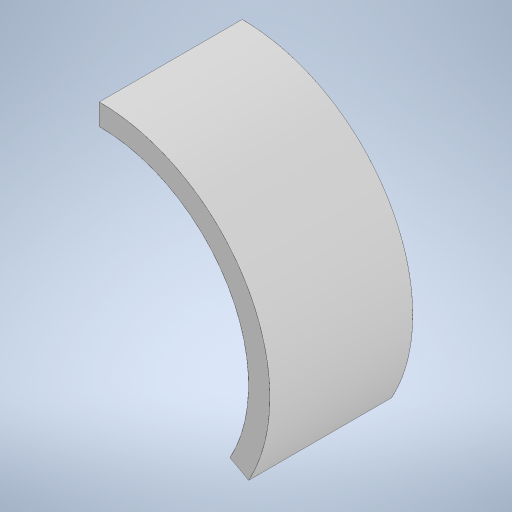
# Autodesk Inventor part: formav2
Saved by Autodesk Inventor 2024 (Build 280153000, 153)
## iProperties
Created: 2023-10-06
Part Number: formav2
Material: Ogólny
Document SubType Name: Modeling
Designer: Pawel
Density: 1 g/cm^3
Appearance: Domyślna
Author: Pawel
Autodesk Inventor part; units mm, degrees
ref_plane "YZ Plane" through (0, 0, 0) normal (1, 0, 0) x (0, 1, 0)
ref_plane "XZ Plane" through (0, 0, 0) normal (0, 1, 0) x (-1, 0, 0)
ref_plane "XY Plane" through (0, 0, 0) normal (0, 0, 1) x (1, 0, 0)
sketch "Szkic1" plane through (0, 0, 0) normal (0, 0, 1) x (1, 0, 0)
  circle A0 centre (0, 0) radius 12
  line L0 (-0.9273, 2.8531) -> (-2, 9.798)
  line L1 (0, 7) -> (0, 5.5022)
  line L2 (0.9273, 2.8531) -> (2, 9.798)
  line L3 (-1.3944, 1.0574) -> (1.3944, 1.0574)
  line L4 (-0.5425, -1.6638) -> (-1.0104, -2.8247)
  line L5 (0.5425, -1.6638) -> (1.0104, -2.8247)
  line L6 (-2.9345, -0.6234) -> (-9.4853, -3.1669)
  line L7 (-2.0072, -2.2296) -> (-7.4853, -6.631)
  line L8 (2.0072, -2.2296) -> (7.4853, -6.631)
  line L9 (2.9345, -0.6234) -> (9.4853, -3.1669)
  arc A1 (-2.0072, -2.2296) -> (-1.0104, -2.8247) centre (0, 0) ccw
  arc A2 (1.0104, -2.8247) -> (2.0072, -2.2296) centre (0, 0) ccw
  arc A3 (2.9345, -0.6234) -> (0.9273, 2.8531) centre (0, 0) ccw
  arc A4 (-0.9273, 2.8531) -> (-2.9345, -0.6234) centre (0, 0) ccw
  arc A5 (-2, 9.798) -> (-9.4853, -3.1669) centre (0, 0) ccw
  arc A6 (-7.4853, -6.631) -> (7.4853, -6.631) centre (0, 0) ccw
  arc A7 (9.4853, -3.1669) -> (2, 9.798) centre (0, 0) ccw
  arc A8 (0.5425, -1.6638) -> (1.3944, 1.0574) centre (0, 0) ccw
  arc A9 (-1.3944, 1.0574) -> (-0.5425, -1.6638) centre (0, 0) ccw
  circle A10 centre (0, 0) radius 13.5
  circle A11 centre (0, 0) radius 14.5
  line L10 (7.4853, -6.631) -> (9.4853, -3.1669)
  line L11 (11.8024, -6.5538) -> (12.6981, -7.0006)
  line L12 (11.8024, -6.5538) -> (0, 0)
  line L13 (0, 0) -> (0, 14.5)
  point P0 (-0.7322, 1.5895)
  point P1 (0.7322, 1.5895)
  point P2 (0, 13.5)
  point P3 (0, 1.0574)
  point P4 (1.5299, -0.8496)
  dimension "d2" = 360
  constraints: 28 end point, 20 point on circle, 11 centre point, 6 coincident, 2 symmetric about line, 2 vertical, 1 horizontal, 22 other
extrude "Wyciągnięcie proste2" add sketch "Szkic1" along normal blind 2 contours L2 A7 L9 A3
extrude "Wyciągnięcie proste3" add sketch "Szkic1" along normal blind 12 contours L13 A11 L11 A10 picked at (13.9327, 2.0769)
extrude "Wyciągnięcie proste4" add sketch "Szkic1" against normal blind 1 contours A0 L12 A8 L3 L13 L1 | A0 L13 A10 L12 | L13 A11 L11 A10 | L2 A7 L9 A3 picked at (12.8872, 1.0013) picked at (13.9327, 2.0769)
thicken "Pogrubienie1" operation add thickness 0.1 both sides no extend neighbours no toward (0.8451894, 0.5344669, 0) faces at (8.4519, 5.3447, 1.3333)
thicken "Pogrubienie2" operation add thickness 0.1 both sides no extend neighbours no toward (-0.3619484, -0.9321981, 0) faces at (5.1181, -1.4713, 0.6667)
thicken "Pogrubienie3" operation add thickness 0.1 both sides no extend neighbours no toward (-0.9882815, 0.1526425, 0) faces at (1.6424, 7.483, 0.6667)
sketch "Szkic2" plane through (0, 0, 0) normal (0, 0, 1) x (1, 0, 0)
  circle A0 centre (0, 0) radius 3
  constraints: 1 centre point, 1 coincident
extrude "Wyciągnięcie proste5" cut sketch "Szkic2" against normal blind 1
thicken "Pogrubienie4" operation cut thickness 1 both sides no extend neighbours no toward (0, 0, 1) faces at (7.6782, 0.304, 2)
sketch "Szkic3" plane through (0, 0, 2) normal (0, 0, 1) x (1, 0, 0)
  arc A0 (2.9345, -0.6234) -> (0.9273, 2.8531) centre (0, 0) ccw projected
  circle A1 centre (0, 0) radius 11.4018
  point P0 (0, 0)
  constraints: 1 centre point, 1 coincident
extrude "Wyciągnięcie proste6" cut sketch "Szkic3" against normal blind 1
fillet "Zaokrąglenie1" radius 2 2 edges at (9.4853, -3.1669, 0.5) (2, 9.798, 0.5)
sketch "Szkic4" plane through (0, 0, 1) normal (0, 0, 1) x (1, 0, 0)
  circle A0 centre (0, 0) radius 11.1803
  constraints: 1 centre point, 1 coincident
extrude "Wyciągnięcie proste7" cut sketch "Szkic4" against normal blind 0.4
sketch "Szkic5" plane through (0, 0, 0.6) normal (0, 0, 1) x (1, 0, 0)
  circle A0 centre (0, 0) radius 10.1
  circle A1 centre (0, 0) radius 9.9
  dimension "d29" = 19.8
  constraints: 2 centre point, 2 coincident
  measures "d29" diameter of A1
extrude "Wyciągnięcie proste8" cut sketch "Szkic5" against normal blind 0.6
thicken "Pogrubienie5" operation add thickness 1 both sides no extend neighbours no toward (0.8408787, 0.5412236, 0) faces at (12.1927, 7.8477, 3.3333)
thicken "Pogrubienie6" operation cut thickness 0.5 both sides no extend neighbours no toward (-0.9089878, 0.4168227, 0) faces at (12.2713, -5.6271, 8)
sketch "Szkic6" plane through (0, 0, 0.6) normal (0, 0, 1) x (1, 0, 0)
  point P0 (0, 0)
sketch "Szkic7" plane through (0, 0, 0.6) normal (0, 0, 1) x (1, 0, 0)
  point P0 (0, 0)
thicken "Pogrubienie7" operation cut thickness 0.15 both sides no extend neighbours no toward (0.3619484, 0.9321981, 0) faces at (5.0567, -1.5547, 0.4)
thicken "Pogrubienie8" operation cut thickness 0.15 both sides no extend neighbours no toward (0.9882815, -0.1526425, 0) faces at (1.1819, 5.1565, 0.4)
thicken "Pogrubienie9" operation cut thickness 0.1 both sides no extend neighbours no toward (-0.9721243, 0.2344659, 0) faces at (9.624, -2.3212, 0.2)
thicken "Pogrubienie10" operation add thickness 0.5 both sides no extend neighbours no toward (0, 0, 1) faces at (7.4796, 0.3186, 0.6)
thicken "Pogrubienie11" operation cut thickness 0.5 both sides no extend neighbours no toward (0.9089878, -0.4168227, 0) faces at (12.2713, -5.6271, 8)
thicken "Pogrubienie12" operation add thickness 0.5 both sides no extend neighbours no toward (0.8408787, 0.5412236, 0) faces at (13.0336, 8.389, 3.3333)
thicken "Pogrubienie13" operation cut thickness 0.1 both sides no extend neighbours no toward (0.9882815, -0.1526425, 0) faces at (1.6712, 7.3417, 0.3667)
thicken "Pogrubienie14" operation cut thickness 0.1 both sides no extend neighbours no toward (0.3619484, 0.9321981, 0) faces at (7.1937, -2.2235, 0.3667)
thicken "Pogrubienie15" operation cut thickness 0.1 both sides no extend neighbours no toward (-0.9696282, -0.2445835, 0) faces at (9.5024, 2.3969, 0.3667)
thicken "Pogrubienie16" operation add thickness 0.4 both sides no extend neighbours no toward (0, 0, -1) faces at (10.2616, -2.4581, -1)
fillet "Zaokrąglenie2" radius 0.5 4 edges at (9.2516, -2.9153, 0.55) (2.1011, 9.4697, 0.55) (0.9273, 2.8531, 0.55) (2.9345, -0.6234, 0.55)
